Autodesk Inventor part; units mm, degrees
(part 2 of 2)
  spline S112 degree 2 poles (-4.7439, -15.8859) (-5.0553, -16.1724) (-5.4416, -16.1724) knots 0 0 0 1 1 1
  spline S113 degree 2 poles (-5.4416, -16.1724) (-5.621, -16.1724) (-5.9898, -16.0429) (-6.1841, -15.9108) knots 0 0 0 1 2 2 2
  line L120 (-6.1841, -15.9108) -> (-6.1841, -13.7778)
  spline S114 degree 2 poles (-6.1841, -13.7778) (-6.1841, -13.4289) (-6.219, -13.267) (-6.2888, -13.2097) (-6.3436, -13.2097) knots 0 0 0 1 2 3 3 3
  spline S115 degree 2 poles (-6.3436, -13.2097) (-6.4059, -13.2097) (-6.5006, -13.2445) knots 0 0 0 1 1 1
  line L121 (-6.5006, -13.2445) -> (-6.533, -13.1623)
  line L122 (-6.533, -13.1623) -> (-5.9125, -12.9106)
  line L123 (-5.9125, -12.9106) -> (-5.8104, -12.9106)
  line L124 (-5.8104, -12.9106) -> (-5.8104, -14.4082)
  line L125 (-5.8104, -14.5503) -> (-5.8104, -15.7812)
  spline S116 degree 2 poles (-5.8104, -15.7812) (-5.6957, -15.8934) (-5.4515, -16.008) (-5.3245, -16.008) knots 0 0 0 1 2 2 2
  spline S117 degree 2 poles (-5.3245, -16.008) (-5.1201, -16.008) (-4.7688, -15.5594) (-4.7688, -15.1309) knots 0 0 0 1 2 2 2
  spline S118 degree 2 poles (-4.7688, -15.1309) (-4.7688, -14.7347) (-5.1201, -14.311) (-5.3444, -14.311) knots 0 0 0 1 2 2 2
  spline S119 degree 2 poles (-5.3444, -14.311) (-5.464, -14.311) (-5.5811, -14.3708) knots 0 0 0 1 1 1
  spline S120 degree 2 poles (-5.5811, -14.3708) (-5.6708, -14.4157) (-5.8104, -14.5503) knots 0 0 0 1 1 1
  line L126 (-4.1907, -14.0494) -> (-3.2288, -14.0494)
  line L127 (-3.2288, -14.0494) -> (-3.2288, -14.1316)
  line L128 (-3.2288, -14.1316) -> (-3.2762, -14.1316)
  spline S121 degree 2 poles (-3.2762, -14.1316) (-3.3759, -14.1316) (-3.478, -14.2188) (-3.478, -14.2836) knots 0 0 0 1 2 2 2
  spline S122 degree 2 poles (-3.478, -14.2836) (-3.478, -14.3733) (-3.4033, -14.5278) knots 0 0 0 1 1 1
  line L129 (-3.4033, -14.5278) -> (-2.8999, -15.5694)
  line L130 (-2.8999, -15.5694) -> (-2.4414, -14.4282)
  spline S123 degree 2 poles (-2.4414, -14.4282) (-2.404, -14.336) (-2.404, -14.2463) knots 0 0 0 1 1 1
  spline S124 degree 2 poles (-2.404, -14.2463) (-2.404, -14.2064) (-2.419, -14.1864) knots 0 0 0 1 1 1
  spline S125 degree 2 poles (-2.419, -14.1864) (-2.4364, -14.1615) (-2.5137, -14.1316) (-2.6109, -14.1316) knots 0 0 0 1 2 2 2
  line L131 (-2.6109, -14.1316) -> (-2.6109, -14.0494)
  line L132 (-2.6109, -14.0494) -> (-1.9406, -14.0494)
  line L133 (-1.9406, -14.0494) -> (-1.9406, -14.1316)
  spline S126 degree 2 poles (-1.9406, -14.1316) (-2.0253, -14.1416) (-2.115, -14.1939) (-2.1673, -14.2687) knots 0 0 0 1 2 2 2
  spline S127 degree 2 poles (-2.1673, -14.2687) (-2.1873, -14.3011) (-2.2446, -14.4431) knots 0 0 0 1 1 1
  line L134 (-2.2446, -14.4431) -> (-3.0818, -16.4964)
  spline S128 degree 2 poles (-3.0818, -16.4964) (-3.2039, -16.7954) (-3.5976, -17.1019) (-3.7795, -17.1019) knots 0 0 0 1 2 2 2
  spline S129 degree 2 poles (-3.7795, -17.1019) (-3.9116, -17.1019) (-4.0835, -16.9499) (-4.0835, -16.8502) knots 0 0 0 1 2 2 2
  spline S130 degree 2 poles (-4.0835, -16.8502) (-4.0835, -16.7555) (-3.9589, -16.6409) (-3.8518, -16.6409) knots 0 0 0 1 2 2 2
  spline S131 degree 2 poles (-3.8518, -16.6409) (-3.777, -16.6409) (-3.65, -16.6907) knots 0 0 0 1 1 1
  spline S132 degree 2 poles (-3.65, -16.6907) (-3.5578, -16.7231) (-3.5353, -16.7231) knots 0 0 0 1 1 1
  spline S133 degree 2 poles (-3.5353, -16.7231) (-3.4681, -16.7231) (-3.3086, -16.5836) (-3.2288, -16.3842) knots 0 0 0 1 2 2 2
  line L135 (-3.2288, -16.3842) -> (-3.0843, -16.0254)
  line L136 (-3.0843, -16.0254) -> (-3.8244, -14.4755)
  spline S134 degree 2 poles (-3.8244, -14.4755) (-3.8568, -14.4057) (-3.9315, -14.3011) knots 0 0 0 1 1 1
  spline S135 degree 2 poles (-3.9315, -14.3011) (-3.9864, -14.2213) (-4.0237, -14.1939) knots 0 0 0 1 1 1
  spline S136 degree 2 poles (-4.0237, -14.1939) (-4.0761, -14.159) (-4.1907, -14.1316) knots 0 0 0 1 1 1
  line L137 (-4.1907, -14.1316) -> (-4.1907, -14.0494)
  line L138 (0.2024, -13.2271) -> (0.2024, -14.4306)
  line L139 (0.2024, -14.4306) -> (0.8727, -14.4306)
  spline S137 degree 2 poles (0.8727, -14.4306) (1.1344, -14.4306) (1.2216, -14.3509) knots 0 0 0 1 1 1
  spline S138 degree 2 poles (1.2216, -14.3509) (1.3412, -14.2487) (1.3536, -13.9871) knots 0 0 0 1 1 1
  line L140 (1.3536, -13.9871) -> (1.4359, -13.9871)
  line L141 (1.4359, -13.9871) -> (1.4359, -15.0511)
  line L142 (1.4359, -15.0511) -> (1.3536, -15.0511)
  spline S139 degree 2 poles (1.3536, -15.0511) (1.3212, -14.8293) (1.2913, -14.767) knots 0 0 0 1 1 1
  spline S140 degree 2 poles (1.2913, -14.767) (1.249, -14.6873) (1.0646, -14.5976) (0.8727, -14.5976) knots 0 0 0 1 2 2 2
  line L143 (0.8727, -14.5976) -> (0.2024, -14.5976)
  line L144 (0.2024, -14.5976) -> (0.2024, -15.6018)
  spline S141 degree 2 poles (0.2024, -15.6018) (0.2024, -15.8036) (0.2373, -15.8909) (0.3295, -15.9432) (0.4541, -15.9432) knots 0 0 0 1 2 3 3 3
  line L145 (0.4541, -15.9432) -> (0.9724, -15.9432)
  spline S142 degree 2 poles (0.9724, -15.9432) (1.2315, -15.9432) (1.4658, -15.8709) (1.5729, -15.7663) knots 0 0 0 1 2 2 2
  spline S143 degree 2 poles (1.5729, -15.7663) (1.7125, -15.6267) (1.8595, -15.3451) knots 0 0 0 1 1 1
  line L146 (1.8595, -15.3451) -> (1.9492, -15.3451)
  line L147 (1.9492, -15.3451) -> (1.6851, -16.1101)
  line L148 (1.6851, -16.1101) -> (-0.6647, -16.1101)
  line L149 (-0.6647, -16.1101) -> (-0.6647, -16.0279)
  line L150 (-0.6647, -16.0279) -> (-0.5576, -16.0279)
  spline S144 degree 2 poles (-0.5576, -16.0279) (-0.448, -16.0279) (-0.3533, -15.9756) knots 0 0 0 1 1 1
  spline S145 degree 2 poles (-0.3533, -15.9756) (-0.281, -15.9382) (-0.2287, -15.7937) (-0.2287, -15.5694) knots 0 0 0 1 2 2 2
  line L151 (-0.2287, -15.5694) -> (-0.2287, -13.5909)
  spline S146 degree 2 poles (-0.2287, -13.5909) (-0.2287, -13.2994) (-0.286, -13.2321) knots 0 0 0 1 1 1
  spline S147 degree 2 poles (-0.286, -13.2321) (-0.3682, -13.1424) (-0.5576, -13.1424) knots 0 0 0 1 1 1
  line L152 (-0.5576, -13.1424) -> (-0.6647, -13.1424)
  line L153 (-0.6647, -13.1424) -> (-0.6647, -13.0601)
  line L154 (-0.6647, -13.0601) -> (1.6875, -13.0601)
  line L155 (1.6875, -13.0601) -> (1.7199, -13.7304)
  line L156 (1.7199, -13.7304) -> (1.6327, -13.7304)
  spline S148 degree 2 poles (1.6327, -13.7304) (1.5854, -13.4887) (1.4708, -13.3093) (1.3586, -13.262) knots 0 0 0 1 2 2 2
  spline S149 degree 2 poles (1.3586, -13.262) (1.2689, -13.2271) (1.0397, -13.2271) knots 0 0 0 1 1 1
  line L157 (1.0397, -13.2271) -> (0.2024, -13.2271)
  line L158 (2.916, -13.9896) -> (2.916, -16.0603)
  spline S150 degree 2 poles (2.916, -16.0603) (2.916, -16.5886) (2.465, -17.1019) (2.1037, -17.1019) knots 0 0 0 1 2 2 2
  spline S151 degree 2 poles (2.1037, -17.1019) (1.8994, -17.1019) (1.7, -16.9524) (1.7, -16.8751) knots 0 0 0 1 2 2 2
  spline S152 degree 2 poles (1.7, -16.8751) (1.7, -16.7954) (1.8096, -16.6833) (1.8844, -16.6833) knots 0 0 0 1 2 2 2
  spline S153 degree 2 poles (1.8844, -16.6833) (1.9442, -16.6833) (2.004, -16.7132) knots 0 0 0 1 1 1
  spline S154 degree 2 poles (2.004, -16.7132) (2.0414, -16.7281) (2.2607, -16.925) (2.3354, -16.925) knots 0 0 0 1 2 2 2
  spline S155 degree 2 poles (2.3354, -16.925) (2.3902, -16.925) (2.4924, -16.8427) (2.5422, -16.6459) (2.5422, -16.3219) knots 0 0 0 1 2 3 3 3
  line L159 (2.5422, -16.3219) -> (2.5422, -14.8567)
  spline S156 degree 2 poles (2.5422, -14.8567) (2.5422, -14.5179) (2.5223, -14.4207) knots 0 0 0 1 1 1
  spline S157 degree 2 poles (2.5223, -14.4207) (2.5074, -14.3459) (2.4376, -14.2886) (2.3803, -14.2886) knots 0 0 0 1 2 2 2
  spline S158 degree 2 poles (2.3803, -14.2886) (2.318, -14.2886) (2.2283, -14.3235) knots 0 0 0 1 1 1
  line L160 (2.2283, -14.3235) -> (2.1959, -14.2413)
  line L161 (2.1959, -14.2413) -> (2.8188, -13.9896)
  line L162 (2.8188, -13.9896) -> (2.916, -13.9896)
  spline S159 degree 2 poles (2.7217, -12.9106) (2.8188, -12.9106) (2.9534, -13.0452) (2.9534, -13.1424) knots 0 0 0 1 2 2 2
  spline S160 degree 2 poles (2.9534, -13.1424) (2.9534, -13.2371) (2.8188, -13.3716) (2.7217, -13.3716) knots 0 0 0 1 2 2 2
  spline S161 degree 2 poles (2.7217, -13.3716) (2.627, -13.3716) (2.4924, -13.2371) (2.4924, -13.1424) knots 0 0 0 1 2 2 2
  spline S162 degree 2 poles (2.4924, -13.1424) (2.4924, -13.0452) (2.627, -12.9106) (2.7217, -12.9106) knots 0 0 0 1 2 2 2
  spline S163 degree 2 poles (3.8255, -14.8268) (3.823, -15.2853) (4.0473, -15.5445) knots 0 0 0 1 1 1
  spline S164 degree 2 poles (4.0473, -15.5445) (4.2741, -15.8061) (4.5781, -15.8061) knots 0 0 0 1 1 1
  spline S165 degree 2 poles (4.5781, -15.8061) (4.7799, -15.8061) (5.0789, -15.5844) (5.1811, -15.3128) knots 0 0 0 1 2 2 2
  line L163 (5.1811, -15.3128) -> (5.2509, -15.3576)
  spline S166 degree 2 poles (5.2509, -15.3576) (5.2035, -15.6666) (4.75, -16.1724) (4.4061, -16.1724) knots 0 0 0 1 2 2 2
  spline S167 degree 2 poles (4.4061, -16.1724) (4.0348, -16.1724) (3.5066, -15.5943) (3.5066, -15.1084) knots 0 0 0 1 2 2 2
  spline S168 degree 2 poles (3.5066, -15.1084) (3.5066, -14.5802) (4.0498, -13.9896) (4.4585, -13.9896) knots 0 0 0 1 2 2 2
  spline S169 degree 2 poles (4.4585, -13.9896) (4.8048, -13.9896) (5.2509, -14.4456) (5.2509, -14.8268) knots 0 0 0 1 2 2 2
  line L164 (5.2509, -14.8268) -> (3.8255, -14.8268)
  line L165 (3.8255, -14.6973) -> (4.7824, -14.6973)
  spline S170 degree 2 poles (4.7824, -14.6973) (4.7699, -14.5004) (4.7351, -14.4182) knots 0 0 0 1 1 1
  spline S171 degree 2 poles (4.7351, -14.4182) (4.6777, -14.2936) (4.456, -14.1491) (4.3339, -14.1491) knots 0 0 0 1 2 2 2
  spline S172 degree 2 poles (4.3339, -14.1491) (4.147, -14.1491) (3.8505, -14.4381) (3.8255, -14.6973) knots 0 0 0 1 2 2 2
  spline S173 degree 2 poles (6.128, -14.4257) (6.4893, -13.9896) (6.8182, -13.9896) knots 0 0 0 1 1 1
  spline S174 degree 2 poles (6.8182, -13.9896) (6.9852, -13.9896) (7.2269, -14.159) (7.2991, -14.3509) knots 0 0 0 1 2 2 2
  spline S175 degree 2 poles (7.2991, -14.3509) (7.349, -14.4855) (7.349, -14.7646) knots 0 0 0 1 1 1
  line L166 (7.349, -14.7646) -> (7.349, -15.6442)
  spline S176 degree 2 poles (7.349, -15.6442) (7.349, -15.8385) (7.3814, -15.9083) knots 0 0 0 1 1 1
  spline S177 degree 2 poles (7.3814, -15.9083) (7.4063, -15.9656) (7.5159, -16.0279) (7.663, -16.0279) knots 0 0 0 1 2 2 2
  line L167 (7.663, -16.0279) -> (7.663, -16.1101)
  line L168 (7.663, -16.1101) -> (6.6413, -16.1101)
  line L169 (6.6413, -16.1101) -> (6.6413, -16.0279)
  line L170 (6.6413, -16.0279) -> (6.6837, -16.0279)
  spline S178 degree 2 poles (6.6837, -16.0279) (6.8282, -16.0279) (6.9428, -15.9407) (6.9652, -15.856) knots 0 0 0 1 2 2 2
  spline S179 degree 2 poles (6.9652, -15.856) (6.9752, -15.8211) (6.9752, -15.6442) knots 0 0 0 1 1 1
  line L171 (6.9752, -15.6442) -> (6.9752, -14.8019)
  spline S180 degree 2 poles (6.9752, -14.8019) (6.9752, -14.5204) (6.8307, -14.2662) (6.6587, -14.2662) knots 0 0 0 1 2 2 2
  spline S181 degree 2 poles (6.6587, -14.2662) (6.3921, -14.2662) (6.128, -14.5577) knots 0 0 0 1 1 1
  line L172 (6.128, -14.5577) -> (6.128, -15.6442)
  spline S182 degree 2 poles (6.128, -15.6442) (6.128, -15.8535) (6.1529, -15.9033) knots 0 0 0 1 1 1
  spline S183 degree 2 poles (6.1529, -15.9033) (6.1853, -15.9681) (6.2949, -16.0279) (6.4644, -16.0279) knots 0 0 0 1 2 2 2
  line L173 (6.4644, -16.0279) -> (6.4644, -16.1101)
  line L174 (6.4644, -16.1101) -> (5.4402, -16.1101)
  line L175 (5.4402, -16.1101) -> (5.4402, -16.0279)
  line L176 (5.4402, -16.0279) -> (5.4851, -16.0279)
  spline S184 degree 2 poles (5.4851, -16.0279) (5.6446, -16.0279) (5.7542, -15.8684) (5.7542, -15.6442) knots 0 0 0 1 2 2 2
  line L177 (5.7542, -15.6442) -> (5.7542, -14.8792)
  spline S185 degree 2 poles (5.7542, -14.8792) (5.7542, -14.5104) (5.7193, -14.3484) (5.6496, -14.2886) (5.5922, -14.2886) knots 0 0 0 1 2 3 3 3
  spline S186 degree 2 poles (5.5922, -14.2886) (5.5299, -14.2886) (5.4427, -14.3235) knots 0 0 0 1 1 1
  line L178 (5.4427, -14.3235) -> (5.4078, -14.2413)
  line L179 (5.4078, -14.2413) -> (6.0308, -13.9896)
  line L180 (6.0308, -13.9896) -> (6.128, -13.9896)
  line L181 (6.128, -13.9896) -> (6.128, -14.4257)
  line L182 (8.5401, -13.9896) -> (8.5401, -15.6442)
  spline S187 degree 2 poles (8.5401, -15.6442) (8.5401, -15.836) (8.5949, -15.9656) (8.707, -16.0279) (8.8516, -16.0279) knots 0 0 0 1 2 3 3 3
  line L183 (8.8516, -16.0279) -> (8.8516, -16.1101)
  line L184 (8.8516, -16.1101) -> (7.8523, -16.1101)
  line L185 (7.8523, -16.1101) -> (7.8523, -16.0279)
  spline S188 degree 2 poles (7.8523, -16.0279) (8.0018, -16.0279) (8.1065, -15.9706) (8.1663, -15.836) (8.1663, -15.6442) knots 0 0 0 1 2 3 3 3
  line L186 (8.1663, -15.6442) -> (8.1663, -14.8518)
  spline S189 degree 2 poles (8.1663, -14.8518) (8.1663, -14.5179) (8.1464, -14.4182) knots 0 0 0 1 1 1
  spline S190 degree 2 poles (8.1464, -14.4182) (8.1314, -14.3459) (8.0616, -14.2886) (8.0043, -14.2886) knots 0 0 0 1 2 2 2
  spline S191 degree 2 poles (8.0043, -14.2886) (7.942, -14.2886) (7.8523, -14.3235) knots 0 0 0 1 1 1
  line L187 (7.8523, -14.3235) -> (7.8199, -14.2413)
  line L188 (7.8199, -14.2413) -> (8.4404, -13.9896)
  line L189 (8.4404, -13.9896) -> (8.5401, -13.9896)
  spline S192 degree 2 poles (8.3532, -12.9106) (8.4479, -12.9106) (8.5799, -13.0427) (8.5799, -13.1374) knots 0 0 0 1 2 2 2
  spline S193 degree 2 poles (8.5799, -13.1374) (8.5799, -13.2321) (8.4479, -13.3666) (8.3532, -13.3666) knots 0 0 0 1 2 2 2
  spline S194 degree 2 poles (8.3532, -13.3666) (8.2585, -13.3666) (8.1239, -13.2321) (8.1239, -13.1374) knots 0 0 0 1 2 2 2
  spline S195 degree 2 poles (8.1239, -13.1374) (8.1239, -13.0427) (8.256, -12.9106) (8.3532, -12.9106) knots 0 0 0 1 2 2 2
  spline S196 degree 2 poles (9.4571, -14.8268) (9.4546, -15.2853) (9.6788, -15.5445) knots 0 0 0 1 1 1
  spline S197 degree 2 poles (9.6788, -15.5445) (9.9056, -15.8061) (10.2096, -15.8061) knots 0 0 0 1 1 1
  spline S198 degree 2 poles (10.2096, -15.8061) (10.4114, -15.8061) (10.7105, -15.5844) (10.8126, -15.3128) knots 0 0 0 1 2 2 2
  line L190 (10.8126, -15.3128) -> (10.8824, -15.3576)
  spline S199 degree 2 poles (10.8824, -15.3576) (10.8351, -15.6666) (10.3815, -16.1724) (10.0377, -16.1724) knots 0 0 0 1 2 2 2
  spline S200 degree 2 poles (10.0377, -16.1724) (9.6664, -16.1724) (9.1381, -15.5943) (9.1381, -15.1084) knots 0 0 0 1 2 2 2
  spline S201 degree 2 poles (9.1381, -15.1084) (9.1381, -14.5802) (9.6813, -13.9896) (10.09, -13.9896) knots 0 0 0 1 2 2 2
  spline S202 degree 2 poles (10.09, -13.9896) (10.4364, -13.9896) (10.8824, -14.4456) (10.8824, -14.8268) knots 0 0 0 1 2 2 2
  line L191 (10.8824, -14.8268) -> (9.4571, -14.8268)
  line L192 (9.4571, -14.6973) -> (10.4139, -14.6973)
  spline S203 degree 2 poles (10.4139, -14.6973) (10.4015, -14.5004) (10.3666, -14.4182) knots 0 0 0 1 1 1
  spline S204 degree 2 poles (10.3666, -14.4182) (10.3093, -14.2936) (10.0875, -14.1491) (9.9654, -14.1491) knots 0 0 0 1 2 2 2
  spline S205 degree 2 poles (9.9654, -14.1491) (9.7785, -14.1491) (9.482, -14.4381) (9.4571, -14.6973) knots 0 0 0 1 2 2 2
  point P0 (0, 0)
  constraints: 2 other
emboss "Рельеф1" sketch "Эскиз14" operation cut depth 2 direction (0, 0, 1)
sketch "Эскиз15" plane through (0, 0, 0) normal (0, 0, -1) x (-1, 0, 0)
  line L0 (22.8867, 239.3563) -> (22.8867, 242.3563)
  line L1 (22.8867, 242.3563) -> (32.8867, 242.3563)
  line L2 (32.8867, 242.3563) -> (32.8867, 227.1563)
  line L3 (32.8867, 227.1563) -> (22.8867, 227.1563)
  line L4 (22.8867, 227.1563) -> (22.8867, 230.1563)
  line L5 (22.8867, 230.1563) -> (29.8867, 230.1563)
  line L6 (29.8867, 236.3563) -> (29.8867, 239.3563) projected
  line L7 (29.8867, 239.3563) -> (29.8867, 230.1563)
  line L8 (29.8867, 239.3563) -> (22.8867, 239.3563)
  line L9 (29.8867, 179.3563) -> (17.8867, 179.3563) projected
  line L10 (22.8867, 179.3563) -> (22.8867, 182.3563)
  line L11 (22.8867, 182.3563) -> (32.8867, 182.3563)
  line L12 (32.8867, 182.3563) -> (32.8867, 167.032)
  line L13 (32.8867, 167.032) -> (22.8867, 167.032)
  line L14 (22.8867, 167.032) -> (22.8867, 170.032)
  line L15 (22.8867, 170.032) -> (29.8867, 170.032)
  line L16 (29.8867, 176.3563) -> (29.8867, 179.3563) projected
  line L17 (29.8867, 170.032) -> (29.8867, 179.3563)
  line L18 (29.8867, 179.3563) -> (22.8867, 179.3563)
  line L19 (29.8867, 170.1563) -> (17.8867, 170.1563) projected
  line L20 (22.3333, 59.3563) -> (22.3333, 62.3563)
  line L21 (22.3333, 62.3563) -> (32.8867, 62.3563)
  line L22 (32.8867, 62.3563) -> (32.8867, 47.1563)
  line L23 (32.8867, 47.1563) -> (22.3333, 47.1563)
  line L24 (22.3333, 47.1563) -> (22.3333, 50.1563)
  line L25 (22.3333, 50.1563) -> (29.8867, 50.1563)
  line L26 (29.8867, 56.3563) -> (29.8867, 59.3563) projected
  line L27 (29.8867, 50.1563) -> (29.8867, 59.3563)
  line L28 (29.8867, 59.3563) -> (22.3333, 59.3563)
  line L29 (26.8167, 119.3563) -> (14.8167, 119.3563) projected
  line L30 (26.8167, 119.3563) -> (26.8167, 110.1563)
  line L31 (26.8167, 110.1563) -> (19.8167, 110.1563)
  line L32 (19.8167, 110.1563) -> (19.8167, 107.1563)
  line L33 (19.8167, 107.1563) -> (29.8167, 107.1563)
  line L34 (29.8167, 107.1563) -> (29.8167, 122.3563)
  line L35 (29.8167, 122.3563) -> (19.8167, 122.3563)
  line L36 (19.8167, 122.3563) -> (19.8167, 119.3563)
  point P0 (0, 0)
  point P1 (29.8867, 237.8563)
  dimension "d192" = 3
  dimension "d193" = 3
  dimension "d194" = 10
  dimension "d195" = 3
  dimension "d196" = 3
  dimension "d197" = 10
  dimension "d198" = 3
  dimension "d199" = 3
  dimension "d203" = 3
  dimension "d204" = 15.2
  dimension "d208" = 3
  dimension "d212" = 3
  dimension "d213" = 3
  dimension "d214" = 7
  dimension "d215" = 10
  constraints: 62 end point, 15 perpendicular, 6 parallel, 4 equal length, 4 point on line, 3 collinear, 3 vertical, 1 midpoint
  measures "d192" distance of L0.start L0.end
  measures "d193" distance of L3.end L4.end
  measures "d194" distance of L2.end L3.end
  measures "d195" distance of L10.start L10.end
  measures "d196" distance of L13.end L14.end
  measures "d197" distance of L12.end L13.end
  measures "d198" distance from line of L2 point (29.887, 237.856)
  measures "d199" distance between parallel lines of L12 L17
  measures "d203" distance of L20.start L20.end
  measures "d204" distance of L21.end L22.end
  measures "d208" distance between parallel lines of L22 L27
  measures "d212" distance of L35.end L36.end
  measures "d213" distance of L31.end L32.end
  measures "d214" distance of L30.end L31.end
  measures "d215" distance of L34.end L35.end
extrude "Выдавливание12" cut sketch "Эскиз15" against normal blind 10
